Autodesk Inventor part; units mm, degrees
(part 7 of 7)
  arc A631 (-1.8197, 19.5895) -> (-1.9822, 19.9489) centre (-7.7369, 17.1307) ccw projected
  arc A632 (-1.7091, 19.2995) -> (-1.8197, 19.5895) centre (-6.6881, 17.5665) ccw projected
  arc A633 (-1.331, 19.3292) -> (-1.7091, 19.2995) centre (0, 0) ccw projected
  arc A634 (-1.2671, 19.633) -> (-1.331, 19.3292) centre (3.8577, 18.3965) ccw projected
  arc A635 (-1.1629, 20.0133) -> (-1.2671, 19.633) centre (4.9618, 18.1301) ccw projected
  arc A636 (-1.0044, 20.4754) -> (-1.1629, 20.0133) centre (6.0894, 17.7834) ccw projected
  arc A637 (-0.6052, 20.4911) -> (-1.0044, 20.4754) centre (0, 0) ccw projected
  arc A638 (-0.4109, 20.0429) -> (-0.6052, 20.4911) centre (-7.4658, 17.2508) ccw projected
  arc A639 (-0.2771, 19.6719) -> (-0.4109, 20.0429) centre (-6.369, 17.6849) ccw projected
  arc A640 (-0.1896, 19.3741) -> (-0.2771, 19.6719) centre (-5.2892, 18.0371) ccw projected
  arc A641 (0.1896, 19.3741) -> (-0.1896, 19.3741) centre (0, 0) ccw projected
  arc A642 (0.2771, 19.6719) -> (0.1896, 19.3741) centre (5.2892, 18.0371) ccw projected
  line L0 (-18.25, 0) -> (18.25, 0)
  circle A643 centre (0, 0) radius 18.25 projected
  line L1 (0, 18.25) -> (0, -18.25)
  line L2 (-18.25, 0) -> (18.25, 0) construction
  arc A644 (-18.25, 2.5) -> (-18.25, -2.5) centre (-18.25, 0) ccw
  arc A645 (18.25, -2.5) -> (18.25, 2.5) centre (18.25, 0) ccw
  line L3 (0, -18.25) -> (0, 18.25) construction
  arc A646 (-2.5, -18.25) -> (2.5, -18.25) centre (0, -18.25) ccw
  arc A647 (2.5, 18.25) -> (-2.5, 18.25) centre (0, 18.25) ccw
  line L4 (-18.078, 2.5) -> (-18.25, 2.5)
  line L5 (-18.25, -2.5) -> (-18.078, -2.5)
  line L6 (-14.7902, -2.5) -> (-5.4544, -2.5)
  line L7 (-5.4544, 2.5) -> (-14.7902, 2.5)
  line L8 (-2.5, 2.5) -> (-2.5, -2.5)
  line L9 (2.5, 2.5) -> (-2.5, 2.5)
  line L10 (-2.5, -2.5) -> (2.5, -2.5)
  line L11 (2.5, -2.5) -> (2.5, 2.5)
  line L12 (-2.5, -5.4544) -> (-2.5, -14.7902)
  line L13 (-2.5, -18.078) -> (-2.5, -18.25)
  arc A648 (-14.7902, -2.5) -> (-2.5, -14.7902) centre (0, 0) ccw
  line L14 (2.5, -18.25) -> (2.5, -18.078)
  line L15 (2.5, -14.7902) -> (2.5, -5.4544)
  line L16 (5.4544, -2.5) -> (14.7902, -2.5)
  line L17 (18.078, -2.5) -> (18.25, -2.5)
  arc A649 (2.5, -14.7902) -> (14.7902, -2.5) centre (0, 0) ccw
  line L18 (18.25, 2.5) -> (18.078, 2.5)
  line L19 (14.7902, 2.5) -> (5.4544, 2.5)
  line L20 (2.5, 5.4544) -> (2.5, 14.7902)
  line L21 (2.5, 18.078) -> (2.5, 18.25)
  arc A650 (14.7902, 2.5) -> (2.5, 14.7902) centre (0, 0) ccw
  arc A651 (-2.5, 14.7902) -> (-14.7902, 2.5) centre (0, 0) ccw
  line L22 (-2.5, 18.25) -> (-2.5, 18.078)
  line L23 (-2.5, 14.7902) -> (-2.5, 5.4544)
  point P0 (-148.5, -105)
  dimension "d31" = 5
  dimension "d32" = 5
  constraints: 52 end point, 50 parallel, 40 tangent, 20 point on circle, 8 centre point, 4 midpoint, 2 collinear, 1 coincident, 1 horizontal, 1 vertical, 21 other
  measures "d31" diameter of A645
  measures "d32" diameter of A647
extrude "押し出し7" cut sketch "スケッチ11" against normal blind 10 contours A1 L20 A650 L19 | L16 A649 L15 A1 | A1 L7 A651 L23 | L12 A648 L6 A1
fillet "フィレット1" radius 1 8 edges at (133.7098, 102.5, 1.5) (146, 90.2098, 1.5) (151, 90.2098, 1.5) (133.7098, 107.5, 1.5) (146, 119.7902, 1.5) (151, 119.7902, 1.5) (163.2902, 107.5, 1.5) (163.2902, 102.5, 1.5)
fillet "フィレット2" radius 5 8 edges at (151, 110.4544, 1.5) (146, 110.4544, 1.5) (143.0456, 107.5, 1.5) (143.0456, 102.5, 1.5) (146, 99.5456, 1.5) (151, 99.5456, 1.5) (153.9544, 107.5, 1.5) (153.9544, 102.5, 1.5)
sketch "スケッチ12" plane through (148.5, 105, 8) normal (0, 0, 1) x (1, 0, 0)
  circle A0 centre (0, 0) radius 2 projected
  arc A1 (0.5552, 3.8616) -> (0.5094, 3.7241) centre (1.0825, 3.6097) ccw projected
  line L0 (0.5094, 3.7241) -> (0.4405, 3.22) projected
  arc A2 (0.4405, 3.22) -> (-0.4405, 3.22) centre (0, 0) ccw projected
  line L1 (-0.4405, 3.22) -> (-0.5094, 3.7241) projected
  arc A3 (-0.5094, 3.7241) -> (-0.5552, 3.8616) centre (-1.0825, 3.6097) ccw projected
  arc A4 (-0.5552, 3.8616) -> (-0.8556, 4.3042) centre (-2.0633, 3.1615) ccw projected
  arc A5 (-0.8556, 4.3042) -> (-2.0309, 5.0806) centre (-3.1127, 2.1651) ccw projected
  arc A6 (-2.0309, 5.0806) -> (-2.1565, 5.0286) centre (0, 0) ccw projected
  arc A7 (-2.1565, 5.0286) -> (-2.4386, 3.6485) centre (0.6701, 3.732) ccw projected
  arc A8 (-2.4386, 3.6485) -> (-2.338, 3.1232) centre (-0.7765, 3.6944) ccw projected
  arc A9 (-2.338, 3.1232) -> (-2.2731, 2.9935) centre (-1.787, 3.3179) ccw projected
  line L2 (-2.2731, 2.9935) -> (-1.9654, 2.5884) projected
  arc A10 (-1.9654, 2.5884) -> (-2.5884, 1.9654) centre (0, 0) ccw projected
  line L3 (-2.5884, 1.9654) -> (-2.9935, 2.2731) projected
  arc A11 (-2.9935, 2.2731) -> (-3.1232, 2.338) centre (-3.3179, 1.787) ccw projected
  arc A12 (-3.1232, 2.338) -> (-3.6485, 2.4386) centre (-3.6944, 0.7765) ccw projected
  arc A13 (-3.6485, 2.4386) -> (-5.0286, 2.1565) centre (-3.732, -0.6701) ccw projected
  arc A14 (-5.0286, 2.1565) -> (-5.0806, 2.0309) centre (0, 0) ccw projected
  arc A15 (-5.0806, 2.0309) -> (-4.3042, 0.8556) centre (-2.1651, 3.1127) ccw projected
  arc A16 (-4.3042, 0.8556) -> (-3.8616, 0.5552) centre (-3.1615, 2.0633) ccw projected
  arc A17 (-3.8616, 0.5552) -> (-3.7241, 0.5094) centre (-3.6097, 1.0825) ccw projected
  line L4 (-3.7241, 0.5094) -> (-3.22, 0.4405) projected
  arc A18 (-3.22, 0.4405) -> (-3.22, -0.4405) centre (0, 0) ccw projected
  line L5 (-3.22, -0.4405) -> (-3.7241, -0.5094) projected
  arc A19 (-3.7241, -0.5094) -> (-3.8616, -0.5552) centre (-3.6097, -1.0825) ccw projected
  arc A20 (-3.8616, -0.5552) -> (-4.3042, -0.8556) centre (-3.1615, -2.0633) ccw projected
  arc A21 (-4.3042, -0.8556) -> (-5.0806, -2.0309) centre (-2.1651, -3.1127) ccw projected
  arc A22 (-5.0806, -2.0309) -> (-5.0286, -2.1565) centre (0, 0) ccw projected
  arc A23 (-5.0286, -2.1565) -> (-3.6485, -2.4386) centre (-3.732, 0.6701) ccw projected
  arc A24 (-3.6485, -2.4386) -> (-3.1232, -2.338) centre (-3.6944, -0.7765) ccw projected
  arc A25 (-3.1232, -2.338) -> (-2.9935, -2.2731) centre (-3.3179, -1.787) ccw projected
  line L6 (-2.9935, -2.2731) -> (-2.5884, -1.9654) projected
  arc A26 (-2.5884, -1.9654) -> (-1.9654, -2.5884) centre (0, 0) ccw projected
  line L7 (-1.9654, -2.5884) -> (-2.2731, -2.9935) projected
  arc A27 (-2.2731, -2.9935) -> (-2.338, -3.1232) centre (-1.787, -3.3179) ccw projected
  arc A28 (-2.338, -3.1232) -> (-2.4387, -3.6513) centre (-0.7765, -3.6944) ccw projected
  arc A29 (-2.4387, -3.6513) -> (-2.1565, -5.0286) centre (0.6701, -3.732) ccw projected
  arc A30 (-2.1565, -5.0286) -> (-2.0309, -5.0806) centre (0, 0) ccw projected
  arc A31 (-2.0309, -5.0806) -> (-0.8556, -4.3042) centre (-3.1127, -2.1651) ccw projected
  arc A32 (-0.8556, -4.3042) -> (-0.5552, -3.8616) centre (-2.0633, -3.1615) ccw projected
  arc A33 (-0.5552, -3.8616) -> (-0.5094, -3.7241) centre (-1.0825, -3.6097) ccw projected
  line L8 (-0.5094, -3.7241) -> (-0.4405, -3.22) projected
  arc A34 (-0.4405, -3.22) -> (0.4405, -3.22) centre (0, 0) ccw projected
  line L9 (0.4405, -3.22) -> (0.5094, -3.7241) projected
  arc A35 (0.5094, -3.7241) -> (0.5552, -3.8616) centre (1.0825, -3.6097) ccw projected
  arc A36 (0.5552, -3.8616) -> (0.8556, -4.3042) centre (2.0633, -3.1615) ccw projected
  arc A37 (0.8556, -4.3042) -> (2.0309, -5.0806) centre (3.1127, -2.1651) ccw projected
  arc A38 (2.0309, -5.0806) -> (2.1565, -5.0286) centre (0, 0) ccw projected
  arc A39 (2.1565, -5.0286) -> (2.4386, -3.6485) centre (-0.6701, -3.732) ccw projected
  arc A40 (2.4386, -3.6485) -> (2.338, -3.1232) centre (0.7765, -3.6944) ccw projected
  arc A41 (2.338, -3.1232) -> (2.2731, -2.9935) centre (1.787, -3.3179) ccw projected
  line L10 (2.2731, -2.9935) -> (1.9654, -2.5884) projected
  arc A42 (1.9654, -2.5884) -> (2.5884, -1.9654) centre (0, 0) ccw projected
  line L11 (2.5884, -1.9654) -> (2.9935, -2.2731) projected
  arc A43 (2.9935, -2.2731) -> (3.1232, -2.338) centre (3.3179, -1.787) ccw projected
  arc A44 (3.1232, -2.338) -> (3.6485, -2.4386) centre (3.6944, -0.7765) ccw projected
  arc A45 (3.6485, -2.4386) -> (5.0286, -2.1565) centre (3.732, 0.6701) ccw projected
  arc A46 (5.0286, -2.1565) -> (5.0806, -2.0309) centre (0, 0) ccw projected
  arc A47 (5.0806, -2.0309) -> (4.3042, -0.8556) centre (2.1651, -3.1127) ccw projected
  arc A48 (4.3042, -0.8556) -> (3.8616, -0.5552) centre (3.1615, -2.0633) ccw projected
  arc A49 (3.8616, -0.5552) -> (3.7241, -0.5094) centre (3.6097, -1.0825) ccw projected
  line L12 (3.7241, -0.5094) -> (3.22, -0.4405) projected
  arc A50 (3.22, -0.4405) -> (3.22, 0.4405) centre (0, 0) ccw projected
  line L13 (3.22, 0.4405) -> (3.7241, 0.5094) projected
  arc A51 (3.7241, 0.5094) -> (3.8616, 0.5552) centre (3.6097, 1.0825) ccw projected
  arc A52 (3.8616, 0.5552) -> (4.3042, 0.8556) centre (3.1615, 2.0633) ccw projected
  arc A53 (4.3042, 0.8556) -> (5.0806, 2.0309) centre (2.1651, 3.1127) ccw projected
  arc A54 (5.0806, 2.0309) -> (5.0286, 2.1565) centre (0, 0) ccw projected
  arc A55 (5.0286, 2.1565) -> (3.6485, 2.4386) centre (3.732, -0.6701) ccw projected
  arc A56 (3.6485, 2.4386) -> (3.1232, 2.338) centre (3.6944, 0.7765) ccw projected
  arc A57 (3.1232, 2.338) -> (2.9935, 2.2731) centre (3.3179, 1.787) ccw projected
  line L14 (2.9935, 2.2731) -> (2.5884, 1.9654) projected
  arc A58 (2.5884, 1.9654) -> (1.9654, 2.5884) centre (0, 0) ccw projected
  line L15 (1.9654, 2.5884) -> (2.2731, 2.9935) projected
  arc A59 (2.2731, 2.9935) -> (2.338, 3.1232) centre (1.787, 3.3179) ccw projected
  arc A60 (2.338, 3.1232) -> (2.4386, 3.6485) centre (0.7765, 3.6944) ccw projected
  arc A61 (2.4386, 3.6485) -> (2.1565, 5.0286) centre (-0.6701, 3.732) ccw projected
  arc A62 (2.1565, 5.0286) -> (2.0309, 5.0806) centre (0, 0) ccw projected
  arc A63 (2.0309, 5.0806) -> (0.8556, 4.3042) centre (3.1127, 2.1651) ccw projected
  arc A64 (0.8556, 4.3042) -> (0.5552, 3.8616) centre (2.0633, 3.1615) ccw projected
  circle A65 centre (0, 0) radius 6 projected
  circle A66 centre (0, 0) radius 18.25 projected
  line L16 (8.0467, -2.5) -> (13.5554, -2.5) projected
  arc A67 (14.5237, -3.75) -> (13.5554, -2.5) centre (13.5554, -3.5) ccw projected
  arc A68 (3.75, -14.5237) -> (14.5237, -3.75) centre (0, 0) ccw projected
  arc A69 (2.5, -13.5554) -> (3.75, -14.5237) centre (3.5, -13.5554) ccw projected
  line L17 (2.5, -13.5554) -> (2.5, -8.0467) projected
  arc A70 (4.0909, -4.3891) -> (2.5, -8.0467) centre (7.5, -8.0467) ccw projected
  arc A71 (-4.0909, -4.3891) -> (4.0909, -4.3891) centre (0, 0) ccw projected
  arc A72 (-2.5, -8.0467) -> (-4.0909, -4.3891) centre (-7.5, -8.0467) ccw projected
  line L18 (-2.5, -8.0467) -> (-2.5, -13.5554) projected
  arc A73 (-3.75, -14.5237) -> (-2.5, -13.5554) centre (-3.5, -13.5554) ccw projected
  arc A74 (-14.5237, -3.75) -> (-3.75, -14.5237) centre (0, 0) ccw projected
  arc A75 (-13.5554, -2.5) -> (-14.5237, -3.75) centre (-13.5554, -3.5) ccw projected
  line L19 (-13.5554, -2.5) -> (-8.0467, -2.5) projected
  arc A76 (-4.3891, -4.0909) -> (-8.0467, -2.5) centre (-8.0467, -7.5) ccw projected
  arc A77 (-4.3891, 4.0909) -> (-4.3891, -4.0909) centre (0, 0) ccw projected
  arc A78 (-8.0467, 2.5) -> (-4.3891, 4.0909) centre (-8.0467, 7.5) ccw projected
  line L20 (-8.0467, 2.5) -> (-13.5554, 2.5) projected
  arc A79 (-14.5237, 3.75) -> (-13.5554, 2.5) centre (-13.5554, 3.5) ccw projected
  arc A80 (-3.75, 14.5237) -> (-14.5237, 3.75) centre (0, 0) ccw projected
  arc A81 (-2.5, 13.5554) -> (-3.75, 14.5237) centre (-3.5, 13.5554) ccw projected
  line L21 (-2.5, 13.5554) -> (-2.5, 8.0467) projected
  arc A82 (-4.0909, 4.3891) -> (-2.5, 8.0467) centre (-7.5, 8.0467) ccw projected
  arc A83 (4.0909, 4.3891) -> (-4.0909, 4.3891) centre (0, 0) ccw projected
  arc A84 (2.5, 8.0467) -> (4.0909, 4.3891) centre (7.5, 8.0467) ccw projected
  line L22 (2.5, 8.0467) -> (2.5, 13.5554) projected
  arc A85 (3.75, 14.5237) -> (2.5, 13.5554) centre (3.5, 13.5554) ccw projected
  arc A86 (14.5237, 3.75) -> (3.75, 14.5237) centre (0, 0) ccw projected
  arc A87 (13.5554, 2.5) -> (14.5237, 3.75) centre (13.5554, 3.5) ccw projected
  line L23 (13.5554, 2.5) -> (8.0467, 2.5) projected
  arc A88 (4.3891, 4.0909) -> (8.0467, 2.5) centre (8.0467, 7.5) ccw projected
  arc A89 (4.3891, -4.0909) -> (4.3891, 4.0909) centre (0, 0) ccw projected
  arc A90 (8.0467, -2.5) -> (4.3891, -4.0909) centre (8.0467, -7.5) ccw projected
  point P0 (-148.5, -105)
